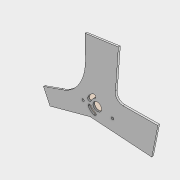
# Autodesk Inventor part: ЛЦМК000002.00.00.00.00.08-01
Saved by Autodesk Inventor 2021.2 (Build 252289000, 289)
## iProperties
Created: 2025-10-27
Part Number: ЛЦМК000002.00.00.00.00.08-01
Material: Типовые
Document SubType Name: Modeling
Designer: Захаров
Density: 1 g/cm^3
Appearance: По умолчанию
Author: Захаров
Autodesk Inventor part; units mm, degrees
ref_plane "YZ Plane" through (0, 0, 0) normal (1, 0, 0) x (0, 1, 0)
ref_plane "XZ Plane" through (0, 0, 0) normal (0, 1, 0) x (-1, 0, 0)
ref_plane "XY Plane" through (0, 0, 0) normal (0, 0, 1) x (1, 0, 0)
ref_plane "РабПлоскость5" through (0, 0, -194) normal (0, 0, 1) x (1, 0, 0)
sketch "Эскиз4" plane through (0, 0, -194) normal (0, 0, 1) x (1, 0, 0)
  line L0 (-7.3772, -14.0792) -> (50, -14.0792)
  line L1 (-60, -33.2323) -> (-7.3772, -14.0792)
  line L2 (-66.8404, -14.4385) -> (-60, -33.2323)
  line L3 (-40.9989, -5.0329) -> (-66.8404, -14.4385)
  arc A0 (-40.9989, -5.0329) -> (-12, 33.9208) centre (-52.4998, 33.7998) ccw
  line L4 (-12, 53.9208) -> (-12, 33.9208)
  line L5 (16, 53.9208) -> (-12, 53.9208)
  line L6 (16, 22.4208) -> (16, 53.9208)
  arc A1 (16, 22.4208) -> (23, 13.9208) centre (23.4314, 21.4084) ccw
  line L7 (50, 13.9208) -> (23, 13.9208)
  line L8 (50, -14.0792) -> (50, 13.9208)
  point P0 (0, 0)
  constraints: 2 centre point, 2 end point
extrude "Выдавливание4" add sketch "Эскиз4" along normal blind 1.8
sketch "Эскиз5" plane through (0, 0, -192.2) normal (0, 0, 1) x (1, 0, 0)
  circle A0 centre (0, 0) radius 4.4
  circle A1 centre (0, 0) radius 12
  circle A2 centre (15, -2) radius 1.2
  line L0 (0, 0) -> (0, -30) construction
  circle A3 centre (-15, -2) radius 1.2
  arc A4 (-3.4374, 7.8273) -> (-8.1316, 2.6381) centre (0, 0) ccw construction
  arc A5 (-4.1781, 9.5141) -> (-9.8839, 3.2066) centre (0, 0) ccw
  arc A6 (-2.6966, 6.1406) -> (-6.3793, 2.0696) centre (0, 0) ccw
  arc A7 (-2.6966, 6.1406) -> (-4.1781, 9.5141) centre (-3.4374, 7.8273) ccw
  arc A8 (-9.8839, 3.2066) -> (-6.3793, 2.0696) centre (-8.1316, 2.6381) ccw
  arc A9 (-7.7059, -3.7016) -> (-2.6966, -8.1124) centre (0, 0) ccw construction
  arc A10 (-9.3665, -4.4992) -> (-3.2777, -9.8605) centre (0, 0) ccw
  arc A11 (-6.0453, -2.9039) -> (-2.1155, -6.3642) centre (0, 0) ccw
  arc A12 (-6.0453, -2.9039) -> (-9.3665, -4.4992) centre (-7.7059, -3.7016) ccw
  arc A13 (-3.2777, -9.8605) -> (-2.1155, -6.3642) centre (-2.6966, -8.1124) ccw
  dimension "d42" = 8.8
  dimension "d43" = 24
  dimension "d44" = 2.4
  dimension "d46" = 30
  dimension "d47" = 15
  dimension "d48" = 2
  constraints: 21 point on circle, 14 centre point, 8 tangent, 4 coincident, 2 concentric, 2 end point, 1 symmetric about line, 1 vertical, 1 other
  measures "d42" diameter of A0
  measures "d43" diameter of A1
  measures "d44" diameter of A2
  measures "d46" distance of L0.start L0.end
  measures "d47" distance from line of L0 A2.centre
  measures "d48" vertical distance of A2.centre point (0, 0)
extrude "Выдавливание5" cut sketch "Эскиз5" against normal blind 30 contours A0 | A2 | A3 | A7 A6 A8 A5 | A12 A11 A13 A10
equation "\"d49\" = d46"
